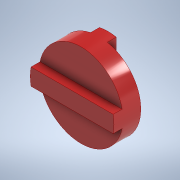
# Autodesk Inventor part: Part1
Saved by Autodesk Inventor 2020 (Build 240168000, 168)
## iProperties
Created: 2021-04-23
Part Number: Part1
Material: Generic
Document SubType Name: Modeling
Designer: Sameer
Density: 1 g/cm^3
Appearance: Red
Author: Sameer
Autodesk Inventor part; units mm, degrees
ref_plane "YZ Plane" through (0, 0, 0) normal (1, 0, 0) x (0, 1, 0)
ref_plane "XZ Plane" through (0, 0, 0) normal (0, 1, 0) x (-1, 0, 0)
ref_plane "XY Plane" through (0, 0, 0) normal (0, 0, 1) x (1, 0, 0)
sketch "Sketch1" plane through (0, 0, 0) normal (0, 0, 1) x (1, 0, 0)
  circle A0 centre (0, 0) radius 75
  line L0 (15, 73.4847) -> (15, -73.4847)
  line L1 (-15, -73.4847) -> (-15, 73.4847)
  dimension "d0" = 150
  dimension "d2" = 15
  constraints: 4 end point, 4 point on circle, 1 centre point, 1 coincident, 1 parallel
  measures "d0" diameter of A0
  measures "d2" distance from line of point (0, 0) L0
extrude "Extrusion1" add sketch "Sketch1" against normal blind 16 contours L0 A0 L1
sketch "Sketch2" plane through (0, 0, 0) normal (0, 0, 1) x (1, 0, 0)
  circle A0 centre (0, 0) radius 75
  constraints: 1 centre point, 1 coincident
extrude "Extrusion2" add sketch "Sketch2" along normal blind 32
sketch "Sketch3" plane through (0, 0, 32) normal (0, 0, 1) x (1, 0, 0)
  line L0 (-75, 15) -> (75, 15)
  line L1 (75, 15) -> (75, -15)
  line L2 (75, -15) -> (-75, -15)
  line L3 (-75, -15) -> (-75, 15)
  point P0 (0, 0)
  dimension "d7" = 30
  dimension "d8" = 15
  dimension "d9" = 75
  dimension "d10" = 75
  constraints: 8 end point, 2 parallel, 1 horizontal, 1 perpendicular
  measures "d7" distance of L2.end L0.start
  measures "d8" distance from line of point (0, 0) L0
  measures "d9" distance from line of point (0, 0) L3
  measures "d10" distance from line of L1 point (0, 0)
extrude "Extrusion3" cut sketch "Sketch3" along normal blind 32
sketch "Sketch4" plane through (0, 0, 32) normal (0, 0, 1) x (1, 0, 0)
  line L0 (-73.4847, 15) -> (73.4847, 15)
  line L1 (73.4847, -15) -> (-73.4847, -15)
  arc A0 (-73.4847, 15) -> (-73.4847, -15) centre (0, 0) ccw
  arc A1 (73.4847, -15) -> (73.4847, 15) centre (0, 0) ccw
  constraints: 4 end point, 4 point on circle, 2 centre point, 1 coincident, 1 horizontal, 1 parallel
extrude "Extrusion4" add sketch "Sketch4" along normal blind 16
equation "\"d2\" = 0.5 * d1"
equation "\"d8\" = 0.5 * d7"
equation "\"d1\" = 30"
body "Solid1"
